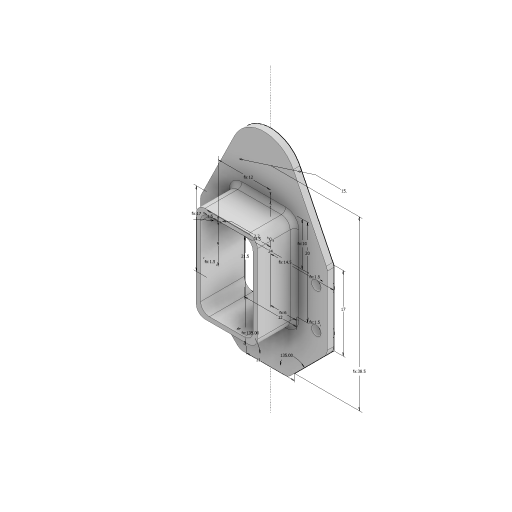
# Autodesk Inventor part: skye_airspeed
Saved by Autodesk Inventor 2023 (Build 270158000, 158)
## iProperties
Created: 2023-06-13
Part Number: skye_airspeed
Material: Generic
Document SubType Name: Modeling
Designer: Thomas
Density: 1 g/cm^3
Appearance: Default
Author: Thomas
Autodesk Inventor part; units mm, degrees
ref_plane "YZ Plane" through (0, 0, 0) normal (1, 0, 0) x (0, 1, 0)
ref_plane "XZ Plane" through (0, 0, 0) normal (0, 1, 0) x (-1, 0, 0)
ref_plane "XY Plane" through (0, 0, 0) normal (0, 0, 1) x (1, 0, 0)
sketch "Sketch1" plane through (0, 0, 0) normal (0, 0, 1) x (1, 0, 0)
  line L0 (-6, 10) -> (6, 10)
  line L1 (6, 10) -> (6, -10)
  line L2 (6, -10) -> (-6, -10)
  line L3 (-6, -10) -> (-6, 10)
  line L4 (-5.5, -21.5) -> (5.5, -21.5)
  line L5 (5.5, -21.5) -> (14.5, -12.5)
  line L6 (14.5, -12.5) -> (14.5, 4.5)
  line L7 (-5.5, -21.5) -> (-14.5, -12.5)
  line L8 (-14.5, -12.5) -> (-14.5, 4.5)
  line L9 (0, -32.2278) -> (0, 36.9858) construction
  circle A0 centre (0, 17) radius 7.5
  line L10 (-14.5, 4.5) -> (-6.731, 20.308)
  line L11 (14.5, 4.5) -> (6.731, 20.308)
  circle A1 centre (-12, 0) radius 1.1
  circle A2 centre (-12, -9) radius 1.1
  circle A3 centre (12, 0) radius 1.1
  circle A4 centre (12, -9) radius 1.1
  line L12 (7, 11) -> (-7, 11)
  line L13 (-7, 11) -> (-7, -11)
  line L14 (-7, -11) -> (7, -11)
  line L15 (7, -11) -> (7, 11)
  circle A5 centre (-12, 0) radius 2.6
  circle A6 centre (-12, -9) radius 2.6
  circle A7 centre (12, 0) radius 2.6
  circle A8 centre (12, -9) radius 2.6
  point P0 (0, 0)
  point P1 (0, -21.5)
  point P2 (0, 2.379)
  dimension "d0" = 12
  dimension "d1" = 20
  dimension "d2" = 10
  dimension "d3" = 6
  dimension "d4" = 11
  dimension "d5" = 21.5
  dimension "d6" = 0
  dimension "d7" = 135
  dimension "d8" = 135
  dimension "d9" = 14.5
  dimension "d10" = 14.5
  dimension "d11" = 15
  dimension "d12" = 38.5
  dimension "d13" = 17
  dimension "d14" = 17
  dimension "d15" = 2.2
  dimension "d18" = 9
  dimension "d21" = 24
  dimension "d24" = 12
  dimension "d25" = 0
  dimension "d30" = 1
  dimension "d34" = 1.5
  dimension "d35" = 1.5
  dimension "d36" = 1.5
  dimension "d37" = 1.5
  constraints: 32 end point, 9 centre point, 4 parallel, 3 horizontal, 3 perpendicular, 3 vertical, 2 midpoint, 2 point on circle, 2 point on line, 2 tangent, 9 other
  measures "d0" distance of L1.end L2.end
  measures "d1" distance of L0.end L1.end
  measures "d2" distance from line of L0 point (0, 0)
  measures "d3" distance from line of L1 point (0, 0)
  measures "d4" distance of L4.start L4.end
  measures "d5" distance from line of point (0, 0) L4
  measures "d6" horizontal distance of point (0, 2.379) point (0, 0)
  measures "d7" angle of L5 L4
  measures "d8" angle of L4 L7
  measures "d9" distance from line of L8 point (0, 0)
  measures "d10" distance from line of L6 point (0, 0)
  measures "d11" diameter of A0
  measures "d12" distance from line of L4 A0.centre
  measures "d13" distance of L5.end L6.end
  measures "d14" distance of L7.end L8.end
  measures "d15" diameter of A1
  measures "d18" distance of A1.centre A2.centre
  measures "d21" distance of A1.centre A3.centre
  measures "d24" distance from line of L9 A1.centre
  measures "d25" vertical distance of point (0, 0) A1.centre
  measures "d30" distance between parallel lines of L0 L12
  measures "d34" radial gap between concentric circles of A1 A5
  measures "d35" radial gap between concentric circles of A2 A6
  measures "d36" radial gap between concentric circles of A3 A7
  measures "d37" radial gap between concentric circles of A4 A8
extrude "Extrusion1" add sketch "Sketch1" along normal blind 1.5 contours L3 L2 L1 L0 A0 L12 L15 L14 L13 | A0 L12 L0 | L12 L13 L14 L15 A0 L11 L6 A7 A8 L5 L4 L7 L8 A6 A5 L10 | A0 L12 | A5 L8 | L6 A7 | A6 L8 | L6 A8 picked at (-14.0333, 0) picked at (14.0333, 0) picked at (-14.0333, -9) picked at (14.0333, -9)
extrude "Extrusion2" add sketch "Sketch1" along normal blind 10 contours L3 L2 L1 L0 A0 L12 L15 L14 L13 | A0 L12 L0
fillet "Fillet1" radius 2 14 edges at (-7, -11, 5.75) (7, -11, 5.75) (7, 11, 5.75) (5.5, -21.5, 0.75) (-5.5, -21.5, 0.75) (14.5, -12.5, 0.75) (-14.5, -12.5, 0.75) (14.5, 4.5, 0.75) (-7, 11, 5.75) (-14.5, 4.5, 0.75) (6, 10, 5) (-6, 10, 5) (-6, -10, 5) (6, -10, 5)
extrude "Extrusion3" [suppressed]
fillet "Fillet2" radius 1 8 edges at (7, 0, 1.5) (6.4142, 10.4142, 1.5) (0, 11, 1.5) (-6.4142, 10.4142, 1.5) (-7, 0, 1.5) (-6.4142, -10.4142, 1.5) (0, -11, 1.5) (6.4142, -10.4142, 1.5)
equation "\"d2\" = 0.5 * d1"
equation "\"d3\" = 0.5 * d0"
equation "\"d8\" = d7"
equation "\"d10\" = d9"
equation "\"d14\" = d13"
equation "\"d24\" = 0.5 * d21"
equation "\"d35\" = d34"
equation "\"d36\" = d34"
equation "\"d37\" = d34"
body "Solid1"
